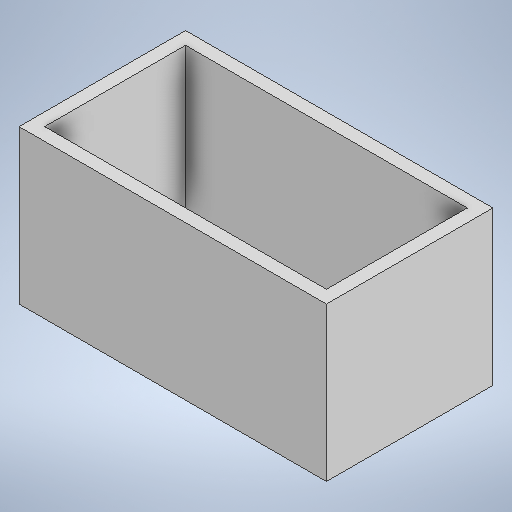
# Autodesk Inventor part: ContraPeso
Saved by Autodesk Inventor 2025 (Build 290162000, 162)
## iProperties
Created: 2025-05-09
Part Number: ContraPeso
Material: Genérico
Document SubType Name: Modeling
Designer: Ian
Density: 1 g/cm^3
Appearance: Padrão
Author: Ian
Autodesk Inventor part; units mm, degrees
ref_plane "YZ Plane" through (0, 0, 0) normal (1, 0, 0) x (0, 1, 0)
ref_plane "XZ Plane" through (0, 0, 0) normal (0, 1, 0) x (-1, 0, 0)
ref_plane "XY Plane" through (0, 0, 0) normal (0, 0, 1) x (1, 0, 0)
sketch "Esboço1" plane through (0, 0, 0) normal (1, 0, 0) x (0, 1, 0)
  line L0 (-30, 32.5) -> (30, 32.5)
  line L1 (30, 32.5) -> (30, -32.5)
  line L2 (30, -32.5) -> (-30, -32.5)
  line L3 (-30, -32.5) -> (-30, 32.5)
  line L4 (-30, 32.5) -> (30, -32.5) construction
  line L5 (30, 32.5) -> (-30, -32.5) construction
  point P0 (0, 0)
  dimension "d0" = 60
  dimension "d1" = 65
  constraints: 12 end point, 2 midpoint, 2 parallel, 1 horizontal, 1 perpendicular
  measures "d0" distance of L1.end L2.end
  measures "d1" distance of L0.end L1.end
extrude "Extrusão1" add sketch "Esboço1" along normal blind 120
sketch "Esboço2" plane through (0, 30, 32.5) normal (0, 1, 0) x (1, 0, 0)
  line L0 (0, 32.5) -> (120, 32.5)
  line L1 (120, 65) -> (120, 0) projected
  line L2 (0, 0) -> (120, 0) projected
  line L3 (60, 0) -> (60, 65)
  line L4 (0, 65) -> (120, 65) projected
  line L5 (115, 5) -> (5, 5)
  line L6 (5, 5) -> (5, 60)
  line L7 (5, 60) -> (115, 60)
  line L8 (115, 60) -> (115, 5)
  line L9 (115, 5) -> (5, 60) construction
  line L10 (5, 5) -> (115, 60) construction
  point P0 (60, 32.5)
  dimension "d4" = 110
  dimension "d5" = 55
  constraints: 16 end point, 6 midpoint, 2 parallel, 1 horizontal, 1 perpendicular
  measures "d4" distance of L6.end L7.end
  measures "d5" distance of L5.end L6.end
extrude "Extrusão2" cut sketch "Esboço2" against normal blind 55 contours L6 L7 L3 L0 | L0 L3 L5 L6 | L3 L7 L8 L0 | L0 L8 L5 L3
